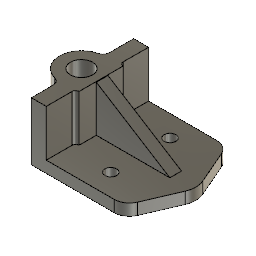
A3 (Autodesk Fusion 360 design; units mm, degrees)
Autodesk Fusion 360 part; units mm, degrees
sketch "Sketch1" plane through (0, 0, 0) normal (0, 0, 1) x (1, 0, 0)
  line L0 (0.467, 42.6724) -> (-58, 42.6724)
  line L1 (-58, -23.151) -> (-58, -45.3276)
  line L2 (-58, -45.3276) -> (0.4398, -45.3276)
  line L3 (9, -45.3276) -> (9, 42.6724)
  line L4 (-58, -1.151) -> (9, -1.151)
  line L5 (9, -1.151) -> (28, -1.151)
  line L6 (12.3821, -37.4639) -> (24.7584, -8.6881)
  line L7 (24.7363, 6.3766) -> (12.3943, 34.8435)
  arc A0 (24.7584, -8.6881) -> (24.7363, 6.3766) centre (7.3042, -1.1812) ccw
  arc A1 (0.4398, -45.3276) -> (12.3821, -37.4639) centre (0.4398, -32.3276) ccw
  arc A2 (12.3943, 34.8435) -> (0.467, 42.6724) centre (0.467, 29.6724) ccw
  line L8 (-55, -1.151) -> (-55, -20.151)
  line L9 (-55, -1.151) -> (-55, 17.849)
  line L10 (-55, -20.151) -> (-55, -20.151)
  line L11 (-55, 17.849) -> (-55, 17.849)
  arc A3 (-55, -20.151) -> (-58, -23.151) centre (-55, -23.151) ccw
  line L12 (-58, 42.6724) -> (-58.1214, 20.8633)
  arc A4 (-58.1214, 20.8633) -> (-55, 17.849) centre (-55.1214, 20.8466) ccw
  line L13 (-58, -45.3276) -> (-71, -45.3276)
  line L14 (-58, 42.6724) -> (-70.9998, 42.7447)
  line L15 (-70.9998, 42.7447) -> (-70.9998, 22.2051)
  arc A5 (-75.5598, 16.3804) -> (-75.56, -20.5089) centre (-70.9998, -2.0642) ccw
  circle A6 centre (-70.9998, -2.0642) radius 9.5
  arc A7 (-75.5598, 16.3804) -> (-70.9998, 22.2051) centre (-76.9998, 22.2051) ccw
  line L16 (-71, -26.3335) -> (-71, -45.3276)
  arc A8 (-71, -26.3335) -> (-75.56, -20.5089) centre (-77, -26.3335) ccw
  circle A9 centre (-21.329, -26.5861) radius 5
  line L17 (9, 42.6724) -> (7.4506, 40.6373) construction
  line L18 (-24.3655, -1.151) -> (-24.5, -1.3276) construction
  line L19 (-24.6345, -1.151) -> (-24.5, -1.3276) construction
  line L20 (7.4417, -43.2809) -> (9, -45.3276) construction
  circle A10 centre (-21.329, 24.2842) radius 5
  point P0 (-58, -20.151)
  dimension "d1" = 67
  dimension "d2" = 88
  dimension "d3" = 19
  dimension "d4" = 19
  dimension "d5" = 13
  dimension "d6" = 13
  dimension "d7" = 19
  dimension "d8" = 3
  dimension "d9" = 3
  dimension "d10" = 3
  dimension "d11" = 13
  dimension "d12" = 13
  dimension "d13" = 38
  dimension "d14" = 19
  dimension "d15" = 6
  dimension "d16" = 6
  dimension "d19" = 10
  constraint horizontal L0
  constraint perpendicular L0 L1
  constraint parallel L0 L2
  constraint parallel L1 L3
  constraint coincident L1 L4.start
  constraint coincident L3 L4.end
  constraint perpendicular L3 L4
  constraint perpendicular L3 L5
  constraint coincident L5.end L7
  constraint coincident L5.end L6
  constraint tangent L7 A0
  constraint tangent L6 A0
  constraint coincident L3.start L2
  constraint coincident L3.start L6
  constraint tangent L2 A1
  constraint tangent L6 A1
  constraint coincident L3.end L0
  constraint coincident L3.end L7
  constraint tangent L0 A2
  constraint tangent L7 A2
  constraint coincident L4 L8.start
  constraint perpendicular L4 L8
  constraint symmetric L4 L8.start L9.start
  constraint symmetric L4 L8.end L9.end
  constraint coincident L1 P0
  constraint coincident L0.end L1
  constraint coincident P0 L10
  constraint tangent L1 A3
  constraint tangent L12 A4
  constraint perpendicular L1 L13
  constraint perpendicular L12 L14
  constraint perpendicular L13 L15
  constraint coincident L15 A5.centre
  constraint concentric A5 A6
  constraint tangent A5 A7
  constraint tangent L15 A7
  constraint perpendicular L13 L16
  constraint tangent A5 A8
  constraint tangent L16 A8
  constraint coincident L4 L19.start
  constraint coincident A2 L17.end
  constraint coincident L4 L18.start
  constraint collinear L17 L18
  constraint coincident A1 L20.start
  constraint collinear L19 L20
  constraint symmetric L4 A9 A10
  measures "d1" distance of L1.end L3.start
  measures "d2" distance of L0.end L1.end
  measures "d3" distance of L4.end L5.end
  measures "d4" radius of A0
  measures "d5" radius of A1
  measures "d6" radius of A2
  measures "d7" distance of L8.start L8.end
  measures "d8" distance of L8.end P0
  measures "d9" radius of A3
  measures "d10" radius of A4
  measures "d11" distance of L1.end L13.end
  measures "d12" distance of L0.end L14.end
  measures "d13" diameter of A5
  measures "d14" diameter of A6
  measures "d15" radius of A7
  measures "d16" radius of A8 L3.end
  measures "d19" diameter of A9
sketch "Sketch2" plane through (0, 0, 0) normal (0, 1, 0) x (1, 0, 0)
  line L0 (-55.7625, -49.9546, -0.3467) -> (-55.7625, 0.0454, -0.3467)
  line L1 (-55.7625, 0.0454, -0.3467) -> (24.2375, 0.0454, -0.3698)
  line L2 (-55.7625, -49.9546, -0.3467) -> (24.2375, 0.0454, -0.3698)
  dimension "d17" = 50
  dimension "d18" = 80
  dimension "d30" = 67
extrude "Extrude1" add sketch "Sketch1" along normal blind 10 contours L0 L3 L4 A2 L9 L12 A4 | L3 L5 L7 A0 A2 | L3 L5 L6 A0 A1 | L1 L2 L3 L4 A1 L8 A3
extrude "Extrude2" add sketch "Sketch1" along normal blind 50 contours L1 L8 L9 A3 L12 A4 L13 L14 L15 A5 A7 L16 A8
extrude "Extrude3" add sketch "Sketch2" along normal mid plane 10 contours L0 L1 L2 in plane through (-0.0001, -0.3628, 0) normal (0.000289, 1, 0)
extrude "Extrude4" add 1 faces at (-62.3333, -31.604, 50) along direction (0, 0, -1) blind 10
